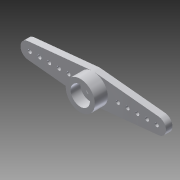
# Autodesk Inventor part: servo arm HK15138 2 cut to 1
Saved by Autodesk Inventor 2013 (Build 170138000, 138)
## iProperties
Created: 2014-06-28
Part Number: servo arm HK15138 2 cut to 1
Material: Generic
Document SubType Name: Modeling
Designer: Masta
Density: 1 g/cm^3
Author: Masta
Autodesk Inventor part; units mm, degrees
ref_plane "YZ Plane" through (0, 0, 0) normal (1, 0, 0) x (0, 1, 0)
ref_plane "XZ Plane" through (0, 0, 0) normal (0, 1, 0) x (-1, 0, 0)
ref_plane "XY Plane" through (0, 0, 0) normal (0, 0, 1) x (1, 0, 0)
sketch "Sketch1" plane through (0, 0, 0) normal (0, 1, 0) x (-1, 0, 0)
  circle A0 centre (0, 0) radius 3
  circle A1 centre (0, 0) radius 4.5
  line L0 (0, 0) -> (7.62, 0) construction
  circle A2 centre (0, 0) radius 1.5
  line L1 (0, 0) -> (0, 4.5) construction
  arc A3 (20.25, -2.4875) -> (20.25, 2.4875) centre (20, 0) ccw
  line L2 (20, 0) -> (0, 0)
  arc A4 (-20.25, 2.4875) -> (-20.25, -2.4875) centre (-20, 0) ccw
  line L3 (20.25, 2.4875) -> (0.45, 4.4774)
  line L4 (20.25, -2.4875) -> (0.45, -4.4774)
  line L5 (-20.25, -2.4875) -> (-0.45, -4.4774)
  line L6 (-20.25, 2.4875) -> (-0.45, 4.4774)
  point P0 (10.62, 0)
  point P1 (13.62, 0)
  point P2 (16.62, 0)
  point P3 (19.62, 0)
  point P4 (-7.62, 0)
  point P5 (-7.62, 0)
  point P6 (-10.62, 0)
  point P7 (-13.62, 0)
  point P8 (-16.62, 0)
  point P9 (-19.62, 0)
  dimension "d0" = 6
  dimension "d1" = 9
  dimension "d2" = 7.62
  dimension "d6" = 3
  dimension "d9" = 3
  dimension "d14" = 2.5
  dimension "d15" = 40
  constraints: 14 end point, 9 point on circle, 9 symmetric about line, 7 tangent, 6 coincident, 5 centre point, 2 horizontal, 1 collinear, 1 perpendicular, 5 other
  measures "d0" diameter of A0
  measures "d1" diameter of A1
  measures "d2" distance of L0.start L0.end
  measures "d6" diameter of A2
  measures "d9" distance of point (7.62, 0) point (10.62, 0)
  measures "d14" radius of A4
  measures "d15" distance of L2.start A4.centre
extrude "Extrusion1" add sketch "Sketch1" along normal blind 2 contours A1 | A1 L3 A3 L4 | A1 L5 A4 L6
extrude "Extrusion2" add sketch "Sketch1" against normal blind 1 contours A0 | A1
extrude "Extrusion3" add sketch "Sketch1" against normal blind 4 contours A1
hole "Hole1" at (-7.62, 0, 0) at (-10.62, 0, 0) at (-13.62, 0, 0) at (-16.62, 0, 0) at (-19.62, 0, 0) at (19.62, 0, 0) at (16.62, 0, 0) at (13.62, 0, 0) at (10.62, 0, 0) at (7.62, 0, 0) direction (0, 1, 0) diameter 1.2 depth 8 tip angle 118
body "Solid1"
